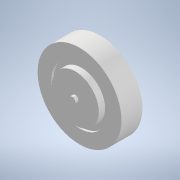
# Autodesk Inventor part: motor at24v
Saved by Autodesk Inventor 2022.2 (Build 262287010, 287A)
## iProperties
Created: 2022-03-16
Part Number: motor at24v
Material: Generic
Document SubType Name: Modeling
Designer: Finn Oriwohl
Density: 1 g/cm^3
Appearance: Default
Author: Finn Oriwohl
Autodesk Inventor part; units mm, degrees
ref_plane "YZ Plane" through (0, 0, 0) normal (1, 0, 0) x (0, 1, 0)
ref_plane "XZ Plane" through (0, 0, 0) normal (0, 1, 0) x (-1, 0, 0)
ref_plane "XY Plane" through (0, 0, 0) normal (0, 0, 1) x (1, 0, 0)
sketch "Sketch1" plane through (0, 0, 0) normal (0, 0, 1) x (1, 0, 0)
  circle A0 centre (0, 0) radius 100
  circle A1 centre (0, 0) radius 56
  circle A2 centre (0, 0) radius 67
  circle A3 centre (0, 0) radius 7.5
  dimension "d0" = 200
  dimension "d1" = 112
  dimension "d2" = 11
  dimension "d3" = 15
  constraints: 4 centre point, 3 coincident
  measures "d0" diameter of A0
  measures "d1" diameter of A1
  measures "d2" radial gap between concentric circles of A1 A2
  measures "d3" diameter of A3
extrude "Extrusion1" add sketch "Sketch1" along normal mid plane 50 contours A0
extrude "Extrusion2" add sketch "Sketch1" along normal mid plane 85 contours A3
extrude "Extrusion3" add sketch "Sketch1" along normal mid plane 70 contours A1
extrude "Extrusion4" add sketch "Sketch1" along normal mid plane 40 contours A2
body "Solid1"
